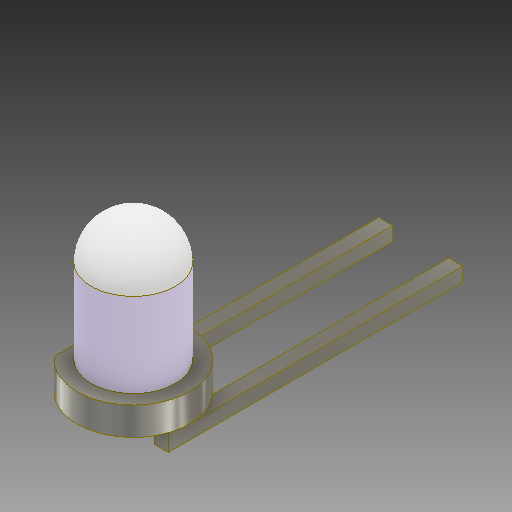
# Autodesk Inventor part: LED 3mm
Saved by Autodesk Inventor 2018 (Build 220112000, 112)
## iProperties
Created: 2019-03-05
Part Number: LED 3mm
Material: Silber
Document SubType Name: Modeling
Designer: RedBots
Density: 10.49 g/cm^3
Appearance: Silber
Mass: 0.476604 g
Surface Area: 1.14984 cm^2
Volume: 0.0454341 cm^3
Author: RedBots
Autodesk Inventor part; units mm, degrees
ref_plane "YZ Plane" through (0, 0, 0) normal (1, 0, 0) x (0, 1, 0)
ref_plane "XZ Plane" through (0, 0, 0) normal (0, 1, 0) x (-1, 0, 0)
ref_plane "XY Plane" through (0, 0, 0) normal (0, 0, 1) x (1, 0, 0)
sketch "Skizze1" plane through (0, 0, 0) normal (0, 0, 1) x (1, 0, 0)
  circle A0 centre (0, 0) radius 1.5
  dimension "d0" = 3
  constraints: 1 centre point, 1 coincident
  measures "d0" diameter of A0
extrude "Extrusion1" add sketch "Skizze1" along normal blind 5.5
fillet "Rundung1" radius 1.5 1 edges at (-1.5, 0, 5.5)
sketch "Skizze2" plane through (0, 0, 0) normal (0, 0, -1) x (-1, 0, 0)
  circle A0 centre (0, 0) radius 2
  line L0 (1.5, 1.3229) -> (1.5, -1.3229)
  circle A1 centre (0, 0) radius 1.5 projected
  point P0 (1.5, 0)
  dimension "d4" = 4
  constraints: 2 end point, 2 point on circle, 1 centre point, 1 coincident, 1 horizontal alignment, 1 midpoint, 1 vertical, 1 other
  measures "d4" diameter of A0
extrude "Extrusion2" add sketch "Skizze2" against normal blind 1 contours L0 A0 picked at (-1.7994, 0.2793)
sketch "Skizze3" plane through (0, 0, 0) normal (0, 0, -1) x (-1, 0, 0)
  line L0 (1.5, -0.25) -> (1, -0.25)
  line L1 (1, -0.25) -> (1, 0.25)
  line L2 (1, 0.25) -> (1.5, 0.25)
  line L3 (1.5, 0.25) -> (1.5, -0.25)
  line L4 (-1, -0.25) -> (-1.5, -0.25)
  line L5 (-1.5, -0.25) -> (-1.5, 0.25)
  line L6 (-1.5, 0.25) -> (-1, 0.25)
  line L7 (-1, 0.25) -> (-1, -0.25)
  line L8 (1, 0) -> (-1, 0) construction
  point P0 (0, 0)
  point P1 (0, 0)
  point P2 (1.25, -0.25)
  point P3 (-1.25, -0.25)
  dimension "d7" = 0.5
  dimension "d9" = 2.5
  constraints: 18 end point, 5 midpoint, 4 parallel, 3 equal length, 2 horizontal, 2 perpendicular, 1 coincident, 1 point on line
  measures "d7" distance of L1.end L2.end
  measures "d9" distance of point (-1.25, -0.25) point (1.25, -0.25)
extrude "Extrusion3" add sketch "Skizze3" along normal blind 1
sketch "Skizze4" plane through (-1.5, 0.25, 0) normal (0, 1, 0) x (1, 0, 0)
  line L0 (0, 0) -> (0, 1) projected
  line L1 (0.5, 0) -> (0.5, 1) projected
  line L2 (0, 1) -> (0.5, 1)
  line L3 (0.5, 1) -> (0.5, 0.5)
  line L4 (0.5, 0.5) -> (0, 0.5)
  line L5 (0, 0.5) -> (0, 1)
  line L6 (2.5, 0) -> (2.5, 1) projected
  line L7 (3, 0) -> (3, 1) projected
  line L8 (2.5, 1) -> (3, 1)
  line L9 (3, 1) -> (3, 0.5)
  line L10 (3, 0.5) -> (2.5, 0.5)
  line L11 (2.5, 0.5) -> (2.5, 1)
  point P0 (1.5, 0)
  constraints: 16 end point, 4 parallel, 2 equal length, 2 horizontal, 2 midpoint, 2 perpendicular
extrude "Extrusion4" add sketch "Skizze4" along normal blind 10
